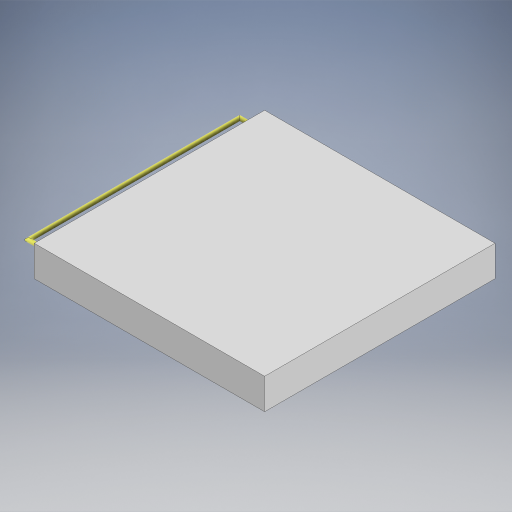
# Autodesk Inventor part: KVA Part Automation
Saved by Autodesk Inventor 2024.2 (Build 282272000, 272)
## iProperties
RuleStatus: InUse
Created: 2024-08-08
Part Number: KVA Part Automation
Material: Generic
Document SubType Name: Modeling
Designer: TiffanyHayden
Density: 1 g/cm^3
Appearance: Default
MODEL: ATQ-60-60-L
Author: TiffanyHayden
Autodesk Inventor part; units mm, degrees
ref_plane "PLANE IN" through (0, 0, 0) normal (0, 0, 1) x (1, 0, 0)
ref_plane "PLANE OUT" through (0, 0, -1524) normal (0, 0, 1) x (1, 0, 0)
ref_plane "PLANE CTR" through (0, 0, 0) normal (1, 0, 0) x (0, 1, 0)
ref_plane "PLANE RH" through (762, 0, 0) normal (1, 0, 0) x (0, 1, 0)
ref_plane "PLANE LH" through (-762, 0, 0) normal (1, 0, 0) x (0, 1, 0)
ref_plane "PLANE TOP" through (0, 0, 0) normal (0, 1, 0) x (-1, 0, 0)
ref_plane "PLANE BOT" through (0, -203.2, 0) normal (0, 1, 0) x (-1, 0, 0)
ref_plane "PLANE HANDLE RH" through (863.6, 0, 0) normal (1, 0, 0) x (0, 1, 0)
ref_plane "PLANE HANDLE LH" through (-863.6, 0, 0) normal (1, 0, 0) x (0, 1, 0)
ref_plane "PLANE HANDLE IN" through (0, 0, -63.5) normal (0, 0, 1) x (1, 0, 0)
ref_plane "PLANE HANDLE OUT" through (0, 0, -1460.5) normal (0, 0, 1) x (1, 0, 0)
ref_plane "PLANE HANDLE TOP" through (0, -63.5, 0) normal (0, 1, 0) x (-1, 0, 0)
sketch "SKETCH BODY" plane through (0, 0, 0) normal (0, 1, 0) x (-1, 0, 0)
  line L0 (762, 0) -> (-762, 0)
  line L1 (-762, 0) -> (-762, -1524)
  line L2 (-762, -1524) -> (762, -1524)
  line L3 (762, -1524) -> (762, 0)
  line L4 (-1066.8, 0) -> (1066.8, 0) projected
  line L5 (-1066.8, -1524) -> (1066.8, -1524) projected
  line L6 (-762, -1828.8) -> (-762, 304.8) projected
  line L7 (762, -1828.8) -> (762, 304.8) projected
  constraints: 8 end point, 4 collinear, 2 parallel, 1 horizontal, 1 perpendicular
extrude "EXT BODY" add sketch "SKETCH BODY" against normal blind 203.2
sketch "SKETCH HANDLE DIA" plane through (762, 0, 0) normal (1, 0, 0) x (0, 1, 0)
  circle A0 centre (-63.5, -63.5) radius 12.7
  line L0 (-63.5, -58.42) -> (-63.5, -93.98) projected
  line L1 (-81.28, -63.5) -> (-45.72, -63.5) projected
  dimension "d14" = 25.4
  constraints: 1 centre point, 1 midpoint, 1 point on line
  measures "d14" diameter of A0
sketch "SKETCH HANDLE PATH" plane through (0, -63.5, 0) normal (0, 1, 0) x (-1, 0, 0)
  line L0 (-863.6, -1722.12) -> (-863.6, 198.12) projected
  line L1 (-853.44, -63.5) -> (-746.76, -63.5) projected
  line L2 (-853.44, -1460.5) -> (-746.76, -1460.5) projected
  line L3 (-762, -63.5) -> (-863.6, -63.5)
  line L4 (-863.6, -63.5) -> (-863.6, -1460.5)
  line L5 (-863.6, -1460.5) -> (-762, -1460.5)
  line L6 (-762, -1460.5) -> (-762, -63.5) construction
  line L7 (-762, -1722.12) -> (-762, 198.12) projected
  constraints: 8 end point, 4 collinear, 2 parallel, 1 horizontal, 1 perpendicular
sweep "SWP HANDLE" add profiles "SKETCH HANDLE DIA" path "SKETCH HANDLE PATH" path curves L3 L4 L5
mirror "MIR HANDLE" about plane through (0, 0, 0) normal (1, 0, 0) remove original yes
equation "\"d12\" = HEIGHT"
equation "\"d1\" = -LENGTH"
equation "\"d2\" = 0.5 * WIDTH"
equation "\"d3\" = -0.5 * WIDTH"
equation "\"d6\" = -HEIGHT"
equation "\"d7\" = HANDLE_OFFSET_CTR"
equation "\"d8\" = -HANDLE_OFFSET_CTR"
equation "\"d9\" = -HANDLE_OFFSET_END"
equation "\"d10\" = -LENGTH + HANDLE_OFFSET_END"
equation "\"d11\" = -HANDLE_OFFSET_TOP"
equation "\"LENGTH\" = 1524"
equation "\"WIDTH\" = 1524"
equation "\"HEIGHT\" = 203.2"
equation "\"HANDLE_GAP\" = 101.6"
equation "\"HANDLE_OFFSET_CTR\" = 0.5 * WIDTH + HANDLE_GAP"
equation "\"HANDLE_OFFSET_END\" = 63.5"
equation "\"HANDLE_OFFSET_TOP\" = 63.5"
body "Solid1"
